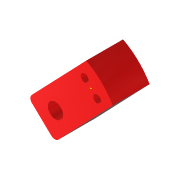
# Autodesk Inventor part: IM_Matchboxscope_Laserholder_M12
Saved by Autodesk Inventor 2022 (Build 260153000, 153)
## iProperties
Created: 2023-05-17
Part Number: IM_Matchboxscope_Laserholder_M12
Material: Generisch
Document SubType Name: Modeling
Designer: diederichbenedict
Density: 1 g/cm^3
Appearance: Glatt - Rot
Author: diederichbenedict
Autodesk Inventor part; units mm, degrees
ref_plane "YZ Plane" through (0, 0, 0) normal (1, 0, 0) x (0, 1, 0)
ref_plane "XZ Plane" through (0, 0, 0) normal (0, 1, 0) x (-1, 0, 0)
ref_plane "XY Plane" through (0, 0, 0) normal (0, 0, 1) x (1, 0, 0)
sketch "Skizze1" plane through (0, 0, 0) normal (0, 0, 1) x (1, 0, 0)
  circle A0 centre (2.503632, -2.442355) radius 1.4 construction
  circle A1 centre (-2.548384, 2.392405) radius 1.4 construction
  arc A2 (8.895275, -1.548845) -> (-1.933457, 8.820314) centre (-14.431862, -15.070948) ccw
  line L0 (-1.933457, 8.820314) -> (-8.895275, 1.545658)
  line L1 (-8.895275, 1.545658) -> (1.936506, -8.820314)
  line L2 (1.936506, -8.820314) -> (8.895275, -1.548845)
  arc A3 (-17.414954, -14.752893) -> (-12.725508, -17.538408) centre (-14.431862, -15.070948) ccw
  line L3 (-8.895275, 1.545658) -> (-25.488913, -15.793637)
  line L4 (-25.488913, -15.793637) -> (-14.657133, -26.159609)
  line L5 (-14.657133, -26.159609) -> (1.936506, -8.820314)
  arc A4 (-13.288846, -12.847547) -> (-12.20846, -16.213964) centre (-14.431862, -15.070948) ccw
  circle A5 centre (-14.431862, -15.070948) radius 3.1
  circle A6 centre (-2.548384, 2.392405) radius 1.6
  circle A7 centre (2.503632, -2.442355) radius 1.6
  circle A8 centre (-22.802017, -23.070943) radius 1.4
  circle A9 centre (-6.057441, -7.070954) radius 1.4
  point P0 (0, 0)
  dimension "d0" = 24
  dimension "d1" = 6.2
  dimension "d2" = 3.2
  dimension "d3" = 3.2
  constraints: 6 end point, 3 centre point, 3 coincident, 2 perpendicular
  measures "d0" distance between parallel lines of L4 L1
  measures "d1" diameter of A5
  measures "d2" diameter of A6
  measures "d3" diameter of A7
extrude "Extrusion1" add sketch "Skizze1" along normal blind 15 contours L2 L1 L0 A2 | L5 L4 L3 L1 | A9
sketch "Skizze2" plane through (0, 0, 15) normal (0, 0, 1) x (1, 0, 0)
  point P0 (0, 0)
sketch "Skizze3" plane through (0, 0, 15) normal (0, 0, 1) x (1, 0, 0)
  point P0 (0, 0)
fillet "Rundung1" radius 2 2 edges at (-14.6571, -26.1596, 7.5) (-25.4889, -15.7936, 7.5)
sketch "Skizze4" plane through (0, 0, 0) normal (0, 0, -1) x (-1, 0, 0)
  circle A0 centre (14.431862, -15.070948) radius 3.1
  line L0 (21.161771, -13.42525) -> (19.222032, -20.076372)
  line L1 (19.222032, -20.076372) -> (12.492123, -21.72207)
  line L2 (12.492123, -21.72207) -> (7.701952, -16.716646)
  line L3 (7.701952, -16.716646) -> (9.641691, -10.065525)
  line L4 (9.641691, -10.065525) -> (16.3716, -8.419827)
  line L5 (16.3716, -8.419827) -> (21.161771, -13.42525)
  line L6 (1.933457, 8.820314) -> (24.10611, -14.348696)
  point P0 (0, 0)
  dimension "d10" = 12
  constraints: 12 end point, 1 coincident, 1 parallel, 13 other
  measures "d10" distance between parallel lines of L2 L5
sketch "Skizze4 outline for Extrusion2" plane through (0, 0, 0) normal (0, 0, -1) x (-1, 0, 0)
  line L0 (21.161771, -13.42525) -> (16.3716, -8.419827)
  line L1 (19.222032, -20.076372) -> (21.161771, -13.42525)
  line L2 (12.492123, -21.72207) -> (19.222032, -20.076372)
  line L3 (7.701952, -16.716646) -> (12.492123, -21.72207)
  line L4 (9.641691, -10.065525) -> (7.701952, -16.716646)
  line L5 (16.3716, -8.419827) -> (9.641691, -10.065525)
extrude "Extrusion2" cut sketch "Skizze4 outline for Extrusion2" against normal blind 5 draft -2
